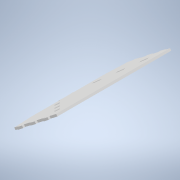
# Autodesk Inventor part: Tolva_Largo
Saved by Autodesk Inventor 2020.1 (Build 241239000, 239)
## iProperties
Created: 2019-12-08
Part Number: Tolva_Largo
Material: Generic
Document SubType Name: Modeling
Designer: Daniel
Density: 1 g/cm^3
Appearance: Default
Author: Daniel
Autodesk Inventor part; units mm, degrees
ref_plane "YZ Plane" through (0, 0, 0) normal (1, 0, 0) x (0, 1, 0)
ref_plane "XZ Plane" through (0, 0, 0) normal (0, 1, 0) x (-1, 0, 0)
sketch "Sketch1" plane through (0, 0, 0) normal (0, 0, 1) x (1, 0, 0)
  line L0 (84, 150) -> (84, -150) projected
  line L1 (-84, 150) -> (-84, -150) projected
  line L2 (-84, 150) -> (84, 150) projected
  line L3 (-15.51, 54.8641) -> (15.51, 54.8641) projected
  line L4 (0, 0) -> (0, 174.1286) construction
  line L5 (15.51, 55.3641) -> (83.5, 108.4837)
  line L6 (15.51, 54.8641) -> (15.51, 55.3641) construction
  line L7 (81.653, 110.8478) -> (13.663, 57.7281)
  line L8 (83.5, 108.4837) -> (81.653, 110.8478)
  line L9 (15.51, 55.3641) -> (13.663, 57.7281)
  line L10 (15.51, 55.3641) -> (0, 55.3641)
  line L11 (13.663, 57.7281) -> (0, 57.7281)
  line L12 (81.653, 110.8478) -> (0, 110.8478)
  line L13 (26.2712, 67.5787) -> (28.1182, 65.2147)
  line L14 (34.1513, 73.7353) -> (35.9983, 71.3713)
  line L15 (53.0636, 88.5112) -> (54.9105, 86.1472)
  line L16 (45.1834, 82.3546) -> (47.0304, 79.9906)
  line L17 (71.9758, 103.2871) -> (73.8228, 100.9231)
  line L18 (64.0957, 97.1305) -> (65.9427, 94.7664)
  dimension "d0" = 0.5
  dimension "d1" = 0.5
  dimension "d2" = 38
  dimension "d3" = 3
  dimension "d4" = 10
  dimension "d5" = 16
  dimension "d8" = 24
  constraints: 33 end point, 5 perpendicular, 5 point on line, 3 vertical, 2 parallel, 14 other
  measures "d0" distance from line of L0 L5.end
  measures "d1" distance from line of L5.start L3
  measures "d2" angle of L5 L3
  measures "d3" distance between parallel lines of L5 L7
  measures "d4" distance between parallel lines of L13 L14
  measures "d5" distance between parallel lines of L9 L13
  measures "d8" distance of L14.start L15.start
extrude "Extrusion1" add sketch "Sketch1" along normal blind 168
sketch "Sketch2" plane through (13.663, 57.7281, 168) normal (-0.6157, 0.788, 0) x (0.788, 0.6157, 0)
  line L0 (-3.8398, 68.49) -> (0, 70.337)
  line L1 (0, 70.337) -> (0, 65.4642)
  line L2 (0, 65.4642) -> (12.5671, 55.5612)
  line L3 (12.5671, 55.5612) -> (14.9359, 58.5673)
  line L4 (14.9359, 58.5673) -> (22.7903, 52.378)
  line L5 (22.7903, 52.378) -> (20.4215, 49.3718)
  line L6 (20.4215, 49.3718) -> (12.5671, 55.5612)
  line L7 (0, 65.4642) -> (-3.8398, 68.49)
  line L8 (20.4215, 49.3718) -> (34.5594, 38.231)
  line L9 (34.5594, 38.231) -> (36.9283, 41.2371)
  line L10 (36.9283, 41.2371) -> (44.7827, 35.0477)
  line L11 (44.7827, 35.0477) -> (42.4138, 32.0416)
  line L12 (42.4138, 32.0416) -> (34.5594, 38.231)
  line L13 (42.4138, 32.0416) -> (56.5518, 20.9008)
  line L14 (56.5518, 20.9008) -> (58.9206, 23.9069)
  line L15 (58.9206, 23.9069) -> (66.775, 17.7175)
  line L16 (66.775, 17.7175) -> (64.4062, 14.7114)
  line L17 (64.4062, 14.7114) -> (56.5518, 20.9008)
  line L18 (64.4062, 14.7114) -> (82.4407, 0.5)
  point P0 (-46.3076, 168)
  constraints: 38 end point, 1 vertical, 34 other
sketch "Sketch4" plane through (83.5, 108.4837, 0) normal (0.6157, -0.788, 0) x (0.788, 0.6157, 0)
  line L0 (-64.3881, 116.7615) -> (-62.0193, 113.7554)
  line L1 (-62.0193, 113.7554) -> (-69.8737, 107.566)
  line L2 (-69.8737, 107.566) -> (-72.2425, 110.5721)
  line L3 (-72.2425, 110.5721) -> (-64.3881, 116.7615)
  line L4 (-42.3958, 134.0917) -> (-40.0269, 131.0856)
  line L5 (-40.0269, 131.0856) -> (-47.8813, 124.8962)
  line L6 (-47.8813, 124.8962) -> (-50.2502, 127.9023)
  line L7 (-50.2502, 127.9023) -> (-42.3958, 134.0917)
  line L8 (-20.4034, 151.4219) -> (-18.0345, 148.4158)
  line L9 (-18.0345, 148.4158) -> (-25.889, 142.2264)
  line L10 (-25.889, 142.2264) -> (-28.2578, 145.2325)
  line L11 (-28.2578, 145.2325) -> (-20.4034, 151.4219)
  point P0 (-132.5881, 0)
  constraints: 24 end point, 24 other
extrude "Extrusion2" cut sketch "Sketch4" against normal blind 10
extrude "Extrusion3" cut sketch "Sketch2" against normal blind 10 contours L14 L15 L16 L17 | L9 L10 L11 L12 | L3 L4 L5 L6
ref_plane "Work Plane1" through (0, 0, 84) normal (0, 0, 1) x (1, 0, 0)
extrude "Extrusion4" add sketch "Sketch1" against normal blind 3 contours L13 L7 L14 L5 | L16 L7 L15 L5 | L18 L7 L17 L5
mirror "Mirror1" about plane through (0, 0, 84) normal (0, 0, 1) of "Extrusion3", "Extrusion2", "Extrusion4"
sketch "Sketch5" plane through (83.5, 108.4837, 0) normal (0.6157, -0.788, 0) x (0.788, 0.6157, 0)
  arc A0 (-87.0927, 88.4093) -> (-87.0927, 79.5907) centre (-115.3496, 84) ccw
  ellipse E0 centre (-105.963, 84) end of major axis (-125.6455, 84) minor radius 15.51 (-87.0927, 88.4093) -> (-92.8236, 95.5479) ccw construction
  arc A1 (-92.8236, 95.5479) -> (-92.8236, 72.4521) centre (-115.3496, 84) ccw construction
  ellipse E1 centre (-105.963, 84) end of major axis (-125.6455, 84) minor radius 15.51 (-92.8236, 72.4521) -> (-87.0927, 79.5907) ccw construction
  ellipse E2 centre (-108.0655, 93.2437) end of major axis (-130.5282, 110.9446) minor radius 17.7588 (-109.3091, 73.4457) -> (-87.7759, 73.4457) ccw projected
  line L0 (-84.8251, 67.3112) -> (-87.7759, 73.4457) projected
  ellipse E3 centre (-108.0655, 74.7563) end of major axis (-130.5282, 57.0554) minor radius 17.7588 (-87.7759, 94.5543) -> (-109.3091, 94.5543) ccw projected
  line L1 (-84.8251, 100.6888) -> (-87.7759, 94.5543) projected
  line L2 (-86.2805, 0) -> (-86.2805, 168) projected
  line L3 (-86.2805, 73.4457) -> (-88.7695, 73.4457)
  line L4 (-86.2805, 94.5543) -> (-88.7695, 94.5543)
  circle A2 centre (-115.3496, 84) radius 28.5989
  point P0 (-132.5881, 0)
  point P1 (-87.0927, 79.5907)
  point P2 (-87.0927, 88.4093)
  constraints: 6 point on circle, 4 end point, 4 point on line, 3 centre point, 1 coincident, 1 concentric, 1 parallel, 1 perpendicular, 20 other
extrude "Extrusion5" add sketch "Sketch5" against normal up to surface (3 mm away) contours A0 L4 L2 L3 A2
chamfer "Chamfer1" distance 30 distance2 8 1 edges at (14.5865, 56.5461, 0) measured on face at (14.2787, 56.9401, 48.9638)
chamfer "Chamfer2" distance 8 distance2 30 1 edges at (14.5865, 56.5461, 168) measured on face at (18.4814, 60.2237, 168)
body "Solid1"
